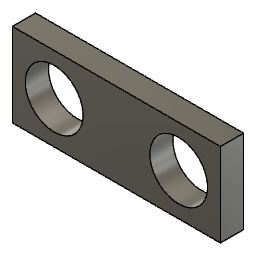
Shooter+piece (Autodesk Fusion 360 design; units mm, degrees)
Autodesk Fusion 360 part; units mm, degrees
sketch "Sketch1" plane through (0, 0, 0) normal (0, 0, 1) x (1, 0, 0) in component "Component"
  line L0 (0, 0) -> (102.743, 0)
  line L1 (102.743, 0) -> (102.743, 41.2496)
  line L2 (102.743, 41.2496) -> (0, 41.2496)
  line L3 (0, 41.2496) -> (0, 0)
  dimension "d1" = 41.2496
  dimension "d10" = 102.743
  constraint horizontal L0
  constraint vertical L1
  constraint horizontal L2
  constraint vertical L3
  constraint coincident L0.start L3.end
  measures "d1" distance of L0.start L2.end
  measures "d10" distance of L1 L3
extrude "Extrude1" add sketch "Sketch1" along normal blind 11.43 in component "Component"
sketch "Sketch2" plane through (0, 0, 11.43) normal (0, 0, 1) x (1, 0, 0) in component "Component"
  line L0 (0, 41.2496) -> (0, 0)
  line L1 (0, 0) -> (102.743, 0)
  line L2 (102.743, 0) -> (102.743, 41.2496)
  line L3 (102.743, 41.2496) -> (0, 41.2496)
  circle A0 centre (20.6248, 20.6248) radius 14.2748
  circle A1 centre (82.1182, 20.6248) radius 14.2748
  dimension "d4" = 28.5496
  dimension "d5" = 28.5496
  dimension "d6" = 20.6248
  dimension "d7" = 20.6248
  dimension "d8" = 20.6248
  dimension "d9" = 61.4934
  measures "d4" diameter of A0
  measures "d5" diameter of A1
  measures "d6" distance of L3 A0.centre
  measures "d7" distance of L1 A1.centre
  measures "d8" distance of L0 A0.centre
  measures "d9" distance of A0.centre A1.centre
extrude "Extrude2" cut sketch "Sketch2" against normal blind 11.43 contours A0 | A1 in component "Component"
component "Component" placed x (1, 0, 0) y (0, 1, 0) z (0, 0, 1) at (0, 0, 0)
